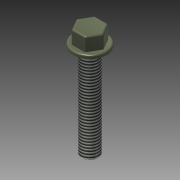
# Autodesk Inventor part: 主动轮护盖固定螺丝
Saved by Autodesk Inventor 2015 (Build 190159000, 159)
## iProperties
Created: 2017-05-12
Part Number: 主动轮护盖固定螺丝
Material: 常规
Document SubType Name: Modeling
Designer: Administrator
Density: 1 g/cm^3
Appearance: 预制平滑
Author: Administrator
Autodesk Inventor part; units mm, degrees
ref_plane "YZ Plane" through (0, 0, 0) normal (1, 0, 0) x (0, 1, 0)
ref_plane "XZ Plane" through (0, 0, 0) normal (0, 1, 0) x (-1, 0, 0)
ref_plane "XY Plane" through (0, 0, 0) normal (0, 0, 1) x (1, 0, 0)
sketch "草图1" plane through (0, 0, 0) normal (0, 0, 1) x (1, 0, 0)
  circle A0 centre (0, 0) radius 5
  dimension "d0" = 10
  constraints: 1 centre point, 1 coincident
  measures "d0" diameter of A0
extrude "拉伸1" add sketch "草图1" along normal blind 1
sketch "草图2" plane through (0, 0, 1) normal (0, 0, 1) x (1, 0, 0)
  line L0 (2.0207, -3.5) -> (-2.0207, -3.5)
  line L1 (-2.0207, -3.5) -> (-4.0415, 0)
  line L2 (-4.0415, 0) -> (-2.0207, 3.5)
  line L3 (-2.0207, 3.5) -> (2.0207, 3.5)
  line L4 (2.0207, 3.5) -> (4.0415, 0)
  line L5 (4.0415, 0) -> (2.0207, -3.5)
  line L6 (0, 0) -> (0, 1.4053)
  circle A0 centre (0, 0) radius 5 projected
  point P0 (0, 3.5)
  dimension "d3" = 1.4053
  dimension "d4" = 3.5
  constraints: 14 end point, 1 coincident, 1 midpoint, 1 point on line, 1 vertical, 13 other
  measures "d3" distance of L6.start L6.end
  measures "d4" distance from line of A0.centre L0
extrude "拉伸2" add sketch "草图2" along normal blind 4 contours L0 L1 L2 L3 L4 L5
fillet "圆角1" radius 0.5 13 edges at (-5, 0, 1) (2.0207, 3.5, 3) (0, 3.5, 5) (-2.0207, 3.5, 3) (-3.0311, 1.75, 5) (-4.0415, 0, 3) (-3.0311, -1.75, 5) (-2.0207, -3.5, 3) (0, -3.5, 5) (2.0207, -3.5, 3) (3.0311, -1.75, 5) (4.0415, 0, 3) (3.0311, 1.75, 5)
sketch "草图3" plane through (0, 0, 0) normal (0, 0, -1) x (-1, 0, 0)
  circle A0 centre (0, 0) radius 2.5
  dimension "d8" = 5
  constraints: 1 centre point, 1 coincident
  measures "d8" diameter of A0
extrude "拉伸3" add sketch "草图3" along normal blind 28
thread "螺纹1" size "M5x0.8" class "6g" standard "ANSI Metric M Profile" full length
chamfer "倒角1" distance 0.25 angle 45 1 edges at (2.5, 0, -28)
